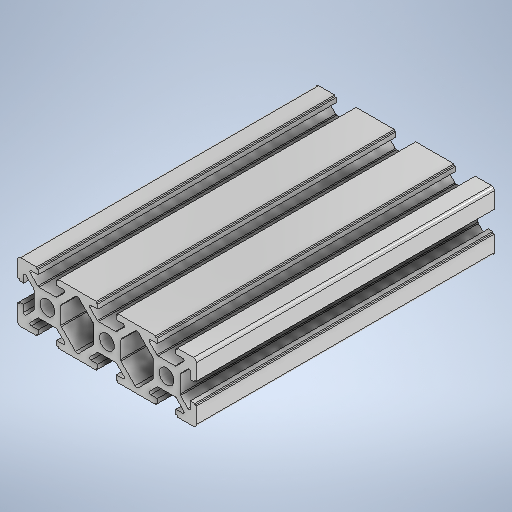
# Autodesk Inventor part: Perfil 20×60 8 rasgos_001
Saved by Autodesk Inventor 2026 (Build 300175000, 175)
## iProperties
Created: 2025-04-01
Part Number: Perfil 20×60 8 rasgos_001
Material: Generic
Document SubType Name: Modeling
Designer: Carlos Dias
Density: 1 g/cm^3
Appearance: Aluminum - Polished
Author: Carlos Dias
Autodesk Inventor part; units mm, degrees
sketch "Sketch2" plane through (0, 0, 0) normal (0, 0, 1) x (1, 0, 0)
  circle A0 centre (0, 0) radius 2.5 construction
  line L0 (-30, 10) -> (0, 10) construction
  arc A1 (0, 2.5) -> (-2.5, 0) centre (0, 0) ccw
  line L1 (-4.5, 4.5) -> (0, 4.5) construction
  line L2 (-4.5, 4.5) -> (-4.5, 0) construction
  line L3 (-9, 9) -> (0, 0) construction
  line L4 (-6.5858, 8) -> (-3.0858, 4.5) construction
  line L5 (-3.1, 8) -> (-6.5858, 8) construction
  line L6 (0, 10) -> (0, 0) construction
  line L7 (-3.1, 10) -> (-3.1, 8) construction
  line L8 (-9.4142, 8) -> (-4.5, 3.0858) construction
  circle A2 centre (-20, 0) radius 2.5 construction
  line L9 (-15.5, 4.5) -> (-15.5, 0) construction
  line L10 (-24.5, 4.5) -> (-15.5, 4.5) construction
  line L11 (-24.5, 4.5) -> (-24.5, 0) construction
  line L12 (-11, 9) -> (-20, 0) construction
  line L13 (-10.5858, 8) -> (-15.5, 3.0858) construction
  line L14 (-13.4142, 8) -> (-16.9142, 4.5) construction
  line L15 (-16.9, 8) -> (-13.4142, 8) construction
  line L16 (-16.9, 10) -> (-16.9, 8) construction
  line L17 (-30, 10) -> (-20, 0) construction
  line L18 (-26.5858, 8) -> (-23.0858, 4.5) construction
  line L19 (-26.5858, 8) -> (-23.1, 8) construction
  line L20 (-23.1, 10) -> (-23.1, 8) construction
  line L21 (-28, 6.5858) -> (-24.5, 3.0858) construction
  line L22 (-30, 10) -> (-30, 0) construction
  line L23 (-28, 6.5858) -> (-28, 3.1) construction
  line L24 (-30, 3.1) -> (-28, 3.1) construction
  arc A3 (-17.5, 0) -> (-22.5, 0) centre (-20, 0) ccw
  arc A4 (-15.3536, 3.2322) -> (-15.5, 2.8787) centre (-15, 2.8787) ccw
  arc A5 (-9.4142, 8) -> (-10.5858, 8) centre (-10, 7.1895) ccw
  arc A6 (-17.1213, 4.5) -> (-16.7678, 4.6464) centre (-17.1213, 5) ccw
  arc A7 (-23.2322, 4.6464) -> (-22.8787, 4.5) centre (-22.8787, 5) ccw
  arc A8 (-24.5, 2.8787) -> (-24.6464, 3.2322) centre (-25, 2.8787) ccw
  arc A9 (-27.1464, 5.7322) -> (-28, 5.3787) centre (-27.5, 5.3787) ccw
  arc A10 (-25.3787, 8) -> (-25.7322, 7.1464) centre (-25.3787, 7.5) ccw
  arc A11 (-14.2678, 7.1464) -> (-14.6213, 8) centre (-14.6213, 7.5) ccw
  arc A12 (-4.5, 2.8787) -> (-4.6464, 3.2322) centre (-5, 2.8787) ccw
  arc A13 (-3.2322, 4.6464) -> (-2.8787, 4.5) centre (-2.8787, 5) ccw
  arc A14 (-5.3787, 8) -> (-5.7322, 7.1464) centre (-5.3787, 7.5) ccw
  line L25 (-30, 3.1) -> (-29.5, 3.1) construction
  line L26 (-29.5, 3.1) -> (-29.5, 3.6)
  line L27 (-29.5, 3.6) -> (-30, 3.6)
  line L28 (-30, 3.6) -> (-30, 3.1) construction
  line L29 (-23.1, 10) -> (-23.6, 10) construction
  line L30 (-23.6, 10) -> (-23.6, 9.5)
  line L31 (-23.6, 9.5) -> (-23.1, 9.5)
  line L32 (-23.1, 9.5) -> (-23.1, 10) construction
  line L33 (-16.9, 10) -> (-16.4, 10) construction
  line L34 (-16.4, 10) -> (-16.4, 9.5)
  line L35 (-16.4, 9.5) -> (-16.9, 9.5)
  line L36 (-16.9, 9.5) -> (-16.9, 10) construction
  line L37 (-3.1, 10) -> (-3.6, 10) construction
  line L38 (-3.6, 10) -> (-3.6, 9.5)
  line L39 (-3.6, 9.5) -> (-3.1, 9.5)
  line L40 (-3.1, 9.5) -> (-3.1, 10) construction
  line L41 (-3.1, 9.5) -> (-3.1, 8)
  line L42 (-5.3787, 8) -> (-3.1, 8)
  line L43 (-16.4, 10) -> (-3.6, 10)
  line L44 (-5.7322, 7.1464) -> (-3.2322, 4.6464)
  line L45 (-2.8787, 4.5) -> (0, 4.5)
  line L46 (0, 4.5) -> (0, 2.5)
  line L47 (-4.5, 0) -> (-2.5, 0)
  line L48 (-4.5, 2.8787) -> (-4.5, 0)
  line L49 (-9.4142, 8) -> (-4.6464, 3.2322)
  line L50 (-10.5858, 8) -> (-15.3536, 3.2322)
  line L51 (-14.2678, 7.1464) -> (-16.7678, 4.6464)
  line L52 (-16.9, 8) -> (-14.6213, 8)
  line L53 (-16.9, 9.5) -> (-16.9, 8)
  line L54 (-15.5, 2.8787) -> (-15.5, 0)
  line L55 (-17.5, 0) -> (-15.5, 0)
  line L56 (-22.8787, 4.5) -> (-17.1213, 4.5)
  line L57 (-24.5, 2.8787) -> (-24.5, 0)
  line L58 (-24.5, 0) -> (-22.5, 0)
  line L59 (-27.1464, 5.7322) -> (-24.6464, 3.2322)
  line L60 (-28, 5.3787) -> (-28, 3.1)
  line L61 (-29.5, 3.1) -> (-28, 3.1)
  line L62 (-30, 9) -> (-30, 3.6)
  arc A15 (-29, 10) -> (-30, 9) centre (-29, 9) ccw
  line L63 (-25.7322, 7.1464) -> (-23.2322, 4.6464)
  line L64 (-25.3787, 8) -> (-23.1, 8)
  line L65 (-23.1, 9.5) -> (-23.1, 8)
  line L66 (-29, 10) -> (-23.6, 10)
  point P0 (0, 5)
  dimension "d74" = 5
  dimension "d76" = 30
  dimension "d78" = 2
  dimension "d79" = 2
  dimension "d80" = 1
  dimension "d82" = 10
  dimension "d83" = 3.1
  dimension "d86" = 1
  dimension "d87" = 20
  dimension "d88" = 2
  dimension "d89" = 2
  dimension "d90" = 1
  dimension "d92" = 2
  dimension "d93" = 1
  dimension "d94" = 3.1
  dimension "d95" = 1
  dimension "d96" = 3.1
  dimension "d97" = 1
  dimension "d98" = 2
  dimension "d99" = 3.1
  dimension "d100" = 0.5
  dimension "d101" = 1
  dimension "d102" = 0.5
  dimension "d103" = 0.5
  dimension "d104" = 0.5
  dimension "d105" = 0.5
  dimension "d106" = 0.5
  dimension "d107" = 0.5
  dimension "d108" = 0.5
  dimension "d109" = 0.5
  dimension "d110" = 0.5
  dimension "d111" = 0.5
  dimension "d113" = 1
  constraints: 134 end point, 33 point on line, 28 point on circle, 24 tangent, 20 horizontal, 16 centre point, 16 vertical, 14 parallel, 12 horizontal alignment, 9 equal length, 6 coincident, 4 perpendicular, 4 vertical alignment, 3 midpoint, 1 equal radius
  measures "d74" diameter of A0
  measures "d76" distance of L0.end L0.start
  measures "d78" distance from line of L46.end L1
  measures "d79" distance from line of L47.end L2
  measures "d80" distance between parallel lines of L3 L4
  measures "d82" distance of L0.end L6.end
  measures "d83" distance from line of L6 L5.start
  measures "d86" distance between parallel lines of L3 L8
  measures "d87" distance of A0.centre A2.centre
  measures "d88" distance edge to line of A2 L9
  measures "d89" distance edge to line of A2 L11
  measures "d90" distance between parallel lines of L12 L13
  measures "d92" distance between parallel lines of L0 L5
  measures "d93" distance between parallel lines of L12 L14
  measures "d94" horizontal distance of A2.centre L15.start
  measures "d95" distance between parallel lines of L17 L18
  measures "d96" horizontal distance of A2.centre L19.end
  measures "d97" distance between parallel lines of L17 L21
  measures "d98" distance from line of L22 L21.start
  measures "d99" vertical distance of A2.centre L23.end
  measures "d100" radius of A4
  measures "d101" radius of A5
  measures "d102" radius of A6
  measures "d103" radius of A7
  measures "d104" radius of A8
  measures "d105" radius of A9
  measures "d106" radius of A10
  measures "d107" radius of A11
  measures "d108" radius of A12
  measures "d109" radius of A13
  measures "d110" radius of A14
  measures "d111" distance of L26.end L27.end
  measures "d113" radius of A15
extrude "Extrusion2" add sketch "Sketch2" along normal mid plane 100
mirror "Mirror1" about plane through (0, 0, 0) normal (0, 1, 0) of "Extrusion2"
mirror "Mirror2" about plane through (0, 0, 0) normal (1, 0, 0) of "Extrusion2", "Mirror1"
equation "\"d79\" = d78"
equation "\"d86\" = d80"
equation "\"d88\" = d78"
equation "\"d89\" = d78"
equation "\"d90\" = d80"
equation "\"d93\" = d80"
equation "\"d94\" = d83"
equation "\"d95\" = d80"
equation "\"d96\" = d83"
body "Solid2"
